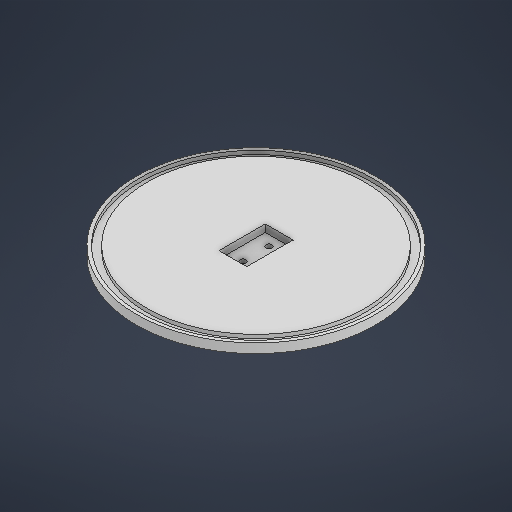
# Autodesk Inventor part: Base_Taza
Saved by Autodesk Inventor 2026 (Build 300175000, 175)
## iProperties
Created: 2025-06-27
Part Number: Base_Taza
Material: Genérico
Document SubType Name: Modeling
Designer: oscar
Density: 1 g/cm^3
Appearance: Valor por defecto
Author: oscar
Autodesk Inventor part; units mm, degrees
ref_plane "YZ Plane" through (0, 0, 0) normal (1, 0, 0) x (0, 1, 0)
ref_plane "XZ Plane" through (0, 0, 0) normal (0, 1, 0) x (-1, 0, 0)
ref_plane "XY Plane" through (0, 0, 0) normal (0, 0, 1) x (1, 0, 0)
sketch "Boceto1" plane through (0, 0, 0) normal (0, 1, 0) x (-1, 0, 0)
  circle A0 centre (0, 0) radius 62.75
  circle A1 centre (0, 0) radius 64.5
  circle A2 centre (0, 0) radius 58.85
  circle A3 centre (0, 0) radius 62.75
  circle A4 centre (0, 0) radius 58.85
  dimension "d0" = 125.5
  dimension "d1" = 129
  dimension "d2" = 117.7
  constraints: 5 centre point, 5 coincident, 2 concentric
  measures "d0" diameter of A0
  measures "d1" diameter of A1
  measures "d2" diameter of A2
extrude "Extrusión1" add sketch "Boceto1" along normal blind 5
sketch "Boceto3" plane through (0, 0, 0) normal (0, -1, 0) x (1, 0, 0)
  circle A0 centre (0, 0) radius 58.85
  circle A1 centre (0, 0) radius 62.75
  constraints: 2 centre point, 2 coincident
extrude "Extrusión2" add sketch "Boceto3" against normal blind 3
sketch "Boceto4" plane through (0, 0, 0) normal (0, -1, 0) x (1, 0, 0)
  line L0 (-7.5, 12.5) -> (7.5, 12.5)
  line L1 (7.5, 12.5) -> (7.5, -12.5)
  line L2 (7.5, -12.5) -> (-7.5, -12.5)
  line L3 (-7.5, -12.5) -> (-7.5, 12.5)
  line L4 (-7.5, 12.5) -> (7.5, -12.5) construction
  line L5 (7.5, 12.5) -> (-7.5, -12.5) construction
  point P0 (0, 0)
  dimension "d7" = 15
  dimension "d8" = 25
  constraints: 12 end point, 2 midpoint, 2 parallel, 1 horizontal, 1 perpendicular
  measures "d7" distance of L1.end L2.end
  measures "d8" distance of L0.end L1.end
extrude "Extrusión3" add sketch "Boceto4" along normal blind 5
sketch "Boceto5" plane through (-7.5, 0, -12.5) normal (-1, 0, 0) x (0, 0, 1)
  line L0 (0, -5) -> (25, -5) projected
  line L1 (25, -5) -> (25, 0)
  line L2 (25, 0) -> (27, 0)
  line L3 (77, 0) -> (-52, 0) projected
  line L4 (27, 0) -> (25, -5)
  line L5 (0, 0) -> (-2, 0)
  line L6 (-2, 0) -> (0, -5)
  line L7 (0, 0) -> (0, -5)
  point P0 (12.5, 0)
  dimension "d11" = 2
  dimension "d12" = 2
  constraints: 12 end point, 3 point on line, 1 perpendicular, 1 vertical
  measures "d11" distance of L1.end L2.end
  measures "d12" distance of L5.start L5.end
extrude "Extrusión4" add sketch "Boceto5" against normal blind 15 contours L6 L3 L7 | L1 L2 L4
sketch "Boceto9" plane through (0, 5, 0) normal (0, 1, 0) x (1, 0, 0)
  line L0 (-7.5, 12.5) -> (7.5, 12.5)
  line L1 (7.5, 12.5) -> (7.5, -12.5)
  line L2 (7.5, -12.5) -> (-7.5, -12.5)
  line L3 (-7.5, -12.5) -> (-7.5, 12.5)
  line L4 (-7.5, 12.5) -> (7.5, -12.5) construction
  line L5 (7.5, 12.5) -> (-7.5, -12.5) construction
  point P0 (0, 0)
  dimension "d15" = 25
  dimension "d16" = 15
  constraints: 12 end point, 2 midpoint, 2 parallel, 1 horizontal, 1 perpendicular
  measures "d15" distance of L0.end L1.end
  measures "d16" distance of L0.start L0.end
extrude "Extrusión5" cut sketch "Boceto9" against normal blind 4
sketch "Boceto10" plane through (0, 1, 0) normal (0, 1, 0) x (1, 0, 0)
  circle A0 centre (0, -7) radius 1.5875
  circle A1 centre (0, 7) radius 1.5875
  point P0 (0, 0)
  dimension "d19" = 3.175
  dimension "d20" = 3.175
  dimension "d21" = 14
  dimension "d22" = 7
  constraints: 2 centre point
  measures "d19" diameter of A0
  measures "d20" diameter of A1
  measures "d21" distance of A1.centre A0.centre
  measures "d22" distance of point (0, 0) A1.centre
extrude "Extrusión6" cut sketch "Boceto10" against normal blind 6
